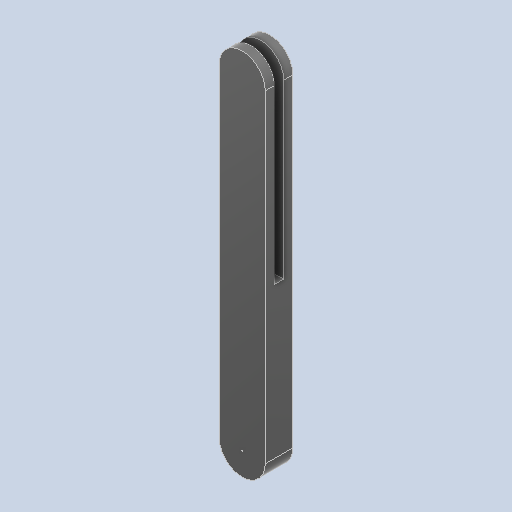
# Autodesk Inventor part: body parts
Saved by Autodesk Inventor 2022 (Build 260153000, 153)
## iProperties
Created: 2022-02-04
Part Number: body parts
Material: PVC-Piping
Document SubType Name: Modeling
Designer: joshw
Density: 1.4 g/cm^3
Appearance: Smooth - Black
Author: joshw
Autodesk Inventor part; units mm, degrees
ref_plane "YZ Plane" through (0, 0, 0) normal (1, 0, 0) x (0, 1, 0)
ref_plane "XZ Plane" through (0, 0, 0) normal (0, 1, 0) x (-1, 0, 0)
ref_plane "XY Plane" through (0, 0, 0) normal (0, 0, 1) x (1, 0, 0)
sketch "Sketch1" plane through (0, 0, 0) normal (0, 0, 1) x (1, 0, 0)
  line L0 (21.0589, 9.4901) -> (21.0589, 9.4901)
  line L1 (21.6939, 8.8551) -> (21.6939, -0.0349)
  line L2 (21.0589, -0.6699) -> (21.0589, -0.6699)
  line L3 (20.4239, -0.0349) -> (20.4239, 8.8551)
  arc A0 (21.0589, 9.4901) -> (20.4239, 8.8551) centre (21.0589, 8.8551) ccw
  arc A1 (21.6939, 8.8551) -> (21.0589, 9.4901) centre (21.0589, 8.8551) ccw
  arc A2 (21.0589, -0.6699) -> (21.6939, -0.0349) centre (21.0589, -0.0349) ccw
  arc A3 (20.4239, -0.0349) -> (21.0589, -0.6699) centre (21.0589, -0.0349) ccw
  point P0 (0, 0)
  point P1 (21.6939, -0.6699)
  point P2 (21.6939, 9.4901)
  point P3 (20.4239, -0.6699)
  dimension "d0" = 1.27
  dimension "d1" = 10.16
  dimension "d2" = 0.635
  constraints: 8 end point, 8 point on circle, 8 tangent, 6 point on line, 4 centre point, 3 equal radius, 2 parallel, 1 horizontal, 1 perpendicular
  measures "d0" distance of point (21.694, -0.67) point (20.424, -0.67)
  measures "d1" distance of point (21.694, 9.49) point (21.694, -0.67)
  measures "d2" radius of A0
extrude "Extrusion1" add sketch "Sketch1" along normal mid plane 0.762
sketch "Sketch2" plane through (0, 0, 0) normal (0, 0, 1) x (1, 0, 0)
  arc A0 (21.6939, 8.8551) -> (20.4239, 8.8551) centre (21.0589, 8.8551) ccw projected
  line L0 (20.4239, 8.8551) -> (20.4239, -0.0349) projected
  line L1 (21.6939, -0.0349) -> (21.6939, 8.8551) projected
  circle A1 centre (21.0589, 8.8551) radius 0.0635
  arc A2 (21.6939, 8.8551) -> (20.4239, 8.8551) centre (21.0589, 8.8551) ccw
  line L2 (20.4239, 4.1124) -> (21.6939, 4.1124)
  line L3 (21.6939, 8.8551) -> (21.6939, -0.0349) projected
  point P0 (0, 0)
  point P1 (20.4239, 8.8551)
  dimension "d5" = 0.127
  constraints: 3 end point, 3 point on line, 2 centre point, 2 coincident, 2 point on circle, 1 perpendicular
  measures "d5" diameter of A1
extrude "Extrusion2" cut sketch "Sketch2" along normal mid plane 0.254
ref_plane "Work Plane1" through (0, 0, 0.127) normal (0, 0, 1) x (1, 0, 0)
sketch "Sketch4" plane through (0, 0, 0.127) normal (0, 0, 1) x (1, 0, 0)
  arc A0 (20.4239, -0.0349) -> (21.6939, -0.0349) centre (21.0589, -0.0349) ccw projected
  circle A1 centre (21.0589, -0.0349) radius 0.0127
  point P0 (0, 0)
  dimension "d11" = 0.0254
  constraints: 1 centre point, 1 coincident
  measures "d11" diameter of A1
extrude "Extrusion4" cut sketch "Sketch4" along normal mid plane 1.8415
body "Solid1"
